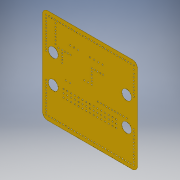
# Autodesk Inventor part: BaseBandAmp_Top_Bottom
Saved by Autodesk Inventor 2018 (Build 220112000, 112)
## iProperties
Created: 2018-03-27
Part Number: BaseBandAmp_Top_Bottom
Material: Generic
Document SubType Name: Modeling
Designer: Eric Weeks
Density: 1 g/cm^3
Appearance: Gold
Author: Eric Weeks
Autodesk Inventor part; units mm, degrees
ref_plane "YZ Plane" through (0, 0, 0) normal (1, 0, 0) x (0, 1, 0)
ref_plane "XZ Plane" through (0, 0, 0) normal (0, 1, 0) x (-1, 0, 0)
ref_plane "XY Plane" through (0, 0, 0) normal (0, 0, 1) x (1, 0, 0)
sketch "Sketch1" plane through (0, 0, 0) normal (0, 0, 1) x (1, 0, 0)
  circle A0 centre (3751.6054, -2038.7056) radius 4.8387 projected
  circle A1 centre (3732.2506, -2038.7056) radius 4.8387 projected
  circle A2 centre (3732.2506, -2038.7056) radius 4.8387 projected
  circle A3 centre (3712.8958, -2038.7056) radius 4.8387 projected
  circle A4 centre (3712.8958, -2038.7056) radius 4.8387 projected
  circle A5 centre (3693.541, -2038.7056) radius 4.8387 projected
  circle A6 centre (3693.541, -2038.7056) radius 4.8387 projected
  circle A7 centre (3674.1862, -2038.7056) radius 4.8387 projected
  circle A8 centre (3674.1862, -2038.7056) radius 4.8387 projected
  circle A9 centre (3751.6054, -2038.7056) radius 4.8387 projected
  line L0 (3839.1338, -1416.8501) -> (3850.1828, -1418.7957) projected
  line L1 (3850.1828, -1418.7957) -> (3850.9956, -1419.098) projected
  line L2 (3850.9956, -1419.098) -> (3860.6984, -1424.6987) projected
  line L3 (3860.6984, -1424.6987) -> (3861.0032, -1424.9425) projected
  line L4 (3861.0032, -1424.9425) -> (3861.3842, -1425.2651) projected
  line L5 (3861.3842, -1425.2651) -> (3868.5724, -1433.8478) projected
  line L6 (3868.5724, -1433.8478) -> (3869.0296, -1434.6123) projected
  line L7 (3869.0296, -1434.6123) -> (3872.865, -1445.1406) projected
  line L8 (3872.865, -1445.1406) -> (3872.9158, -1445.4657) projected
  line L9 (3872.9158, -1445.4657) -> (3872.992, -1445.7883) projected
  line L10 (3872.992, -1445.7883) -> (3873.5, -1451.389) projected
  line L11 (3873.5, -1451.389) -> (3873.4746, -1451.4627) projected
  line L12 (3873.4746, -1451.4627) -> (3873.5, -1451.5541) projected
  line L13 (3873.5, -1451.5541) -> (3873.5, -2032.3099) projected
  line L14 (3873.5, -2032.3099) -> (3873.4492, -2032.5283) projected
  line L15 (3873.4492, -2032.5283) -> (3873.4492, -2032.696) projected
  line L16 (3873.4492, -2032.696) -> (3871.5188, -2043.7272) projected
  line L17 (3871.5188, -2043.7272) -> (3871.214, -2044.5578) projected
  line L18 (3871.214, -2044.5578) -> (3865.6006, -2054.258) projected
  line L19 (3865.6006, -2054.258) -> (3865.0418, -2054.9337) projected
  line L20 (3865.0418, -2054.9337) -> (3856.4566, -2062.1371) projected
  line L21 (3856.4566, -2062.1371) -> (3855.6946, -2062.5765) projected
  line L22 (3855.6946, -2062.5765) -> (3845.179, -2066.4094) projected
  line L23 (3845.179, -2066.4094) -> (3844.8488, -2066.4653) projected
  line L24 (3844.8488, -2066.4653) -> (3844.5186, -2066.5516) projected
  line L25 (3844.5186, -2066.5516) -> (3838.9306, -2067.0418) projected
  line L26 (3838.9306, -2067.0418) -> (3838.8544, -2067.0368) projected
  line L27 (3838.8544, -2067.0368) -> (3838.7528, -2067.052) projected
  line L28 (3838.7528, -2067.052) -> (3258.0072, -2067.052) projected
  line L29 (3258.0072, -2067.052) -> (3257.7786, -2067.0139) projected
  line L30 (3257.7786, -2067.0139) -> (3257.6262, -2067.0139) projected
  line L31 (3257.6262, -2067.0139) -> (3246.5772, -2065.0683) projected
  line L32 (3246.5772, -2065.0683) -> (3245.7644, -2064.766) projected
  line L33 (3245.7644, -2064.766) -> (3236.0616, -2059.1653) projected
  line L34 (3236.0616, -2059.1653) -> (3235.7568, -2058.9215) projected
  line L35 (3235.7568, -2058.9215) -> (3235.3758, -2058.5989) projected
  line L36 (3235.3758, -2058.5989) -> (3228.1876, -2050.0162) projected
  line L37 (3228.1876, -2050.0162) -> (3227.7304, -2049.2517) projected
  line L38 (3227.7304, -2049.2517) -> (3223.895, -2038.7234) projected
  line L39 (3223.895, -2038.7234) -> (3223.8442, -2038.3983) projected
  line L40 (3223.8442, -2038.3983) -> (3223.768, -2038.0757) projected
  line L41 (3223.768, -2038.0757) -> (3223.26, -2032.475) projected
  line L42 (3223.26, -2032.475) -> (3223.2854, -2032.4013) projected
  line L43 (3223.2854, -2032.4013) -> (3223.26, -2032.3099) projected
  line L44 (3223.26, -2032.3099) -> (3223.26, -1451.5541) projected
  line L45 (3223.26, -1451.5541) -> (3223.3108, -1451.3357) projected
  line L46 (3223.3108, -1451.3357) -> (3223.3108, -1451.168) projected
  line L47 (3223.3108, -1451.168) -> (3225.2412, -1440.1368) projected
  line L48 (3225.2412, -1440.1368) -> (3225.546, -1439.3062) projected
  line L49 (3225.546, -1439.3062) -> (3231.1594, -1429.606) projected
  line L50 (3231.1594, -1429.606) -> (3231.4388, -1429.2682) projected
  line L51 (3231.4388, -1429.2682) -> (3231.7182, -1428.9303) projected
  line L52 (3231.7182, -1428.9303) -> (3240.3034, -1421.7269) projected
  line L53 (3240.3034, -1421.7269) -> (3241.0654, -1421.2875) projected
  line L54 (3241.0654, -1421.2875) -> (3251.581, -1417.4546) projected
  line L55 (3251.581, -1417.4546) -> (3251.9112, -1417.3987) projected
  line L56 (3251.9112, -1417.3987) -> (3252.2414, -1417.3124) projected
  line L57 (3252.2414, -1417.3124) -> (3257.8294, -1416.8222) projected
  line L58 (3257.8294, -1416.8222) -> (3257.9056, -1416.8272) projected
  line L59 (3257.9056, -1416.8272) -> (3258.0072, -1416.812) projected
  line L60 (3258.0072, -1416.812) -> (3838.7528, -1416.812) projected
  line L61 (3838.7528, -1416.812) -> (3838.9814, -1416.8501) projected
  line L62 (3838.9814, -1416.8501) -> (3839.1338, -1416.8501) projected
  circle A10 centre (3848.3794, -1470.9648) radius 4.8387 projected
  circle A11 centre (3848.3794, -1470.9648) radius 4.8387 projected
  circle A12 centre (3770.9602, -1445.1584) radius 4.8387 projected
  circle A13 centre (3770.9602, -1445.1584) radius 4.8387 projected
  circle A14 centre (3790.315, -1445.1584) radius 4.8387 projected
  circle A15 centre (3790.315, -1445.1584) radius 4.8387 projected
  circle A16 centre (3809.6698, -1445.1584) radius 4.8387 projected
  circle A17 centre (3809.6698, -1445.1584) radius 4.8387 projected
  circle A18 centre (3848.3794, -1445.1584) radius 4.8387 projected
  circle A19 centre (3848.3794, -1445.1584) radius 4.8387 projected
  circle A20 centre (3829.0246, -1445.1584) radius 4.8387 projected
  circle A21 centre (3829.0246, -1445.1584) radius 4.8387 projected
  circle A22 centre (3848.3794, -1593.5452) radius 4.8387 projected
  circle A23 centre (3848.3794, -1593.5452) radius 4.8387 projected
  circle A24 centre (3848.3794, -1612.9) radius 4.8387 projected
  circle A25 centre (3848.3794, -1612.9) radius 4.8387 projected
  circle A26 centre (3848.3794, -1632.2548) radius 4.8387 projected
  circle A27 centre (3848.3794, -1632.2548) radius 4.8387 projected
  circle A28 centre (3799.9924, -1645.158) radius 33.8709 projected
  circle A29 centre (3777.4118, -1783.8674) radius 4.8387 projected
  circle A30 centre (3799.9924, -1645.158) radius 33.8709 projected
  circle A31 centre (3848.3794, -1574.1904) radius 4.8387 projected
  circle A32 centre (3561.2832, -1606.4484) radius 4.8387 projected
  circle A33 centre (3580.638, -1606.4484) radius 4.8387 projected
  circle A34 centre (3599.9928, -1606.4484) radius 4.8387 projected
  circle A35 centre (3619.3476, -1606.4484) radius 4.8387 projected
  circle A36 centre (3638.7024, -1606.4484) radius 4.8387 projected
  circle A37 centre (3480.6382, -1445.1584) radius 4.8387 projected
  circle A38 centre (3499.993, -1445.1584) radius 4.8387 projected
  circle A39 centre (3635.4766, -1445.1584) radius 4.8387 projected
  circle A40 centre (3635.4766, -1445.1584) radius 4.8387 projected
  circle A41 centre (3616.1218, -1445.1584) radius 4.8387 projected
  circle A42 centre (3616.1218, -1445.1584) radius 4.8387 projected
  circle A43 centre (3638.7024, -1606.4484) radius 4.8387 projected
  circle A44 centre (3635.4766, -1548.384) radius 4.8387 projected
  circle A45 centre (3596.767, -1445.1584) radius 4.8387 projected
  circle A46 centre (3577.4122, -1445.1584) radius 4.8387 projected
  circle A47 centre (3577.4122, -1445.1584) radius 4.8387 projected
  circle A48 centre (3606.4444, -1548.384) radius 4.8387 projected
  circle A49 centre (3558.0574, -1445.1584) radius 4.8387 projected
  circle A50 centre (3558.0574, -1445.1584) radius 4.8387 projected
  circle A51 centre (3577.4122, -1548.384) radius 4.8387 projected
  circle A52 centre (3548.38, -1548.384) radius 4.8387 projected
  circle A53 centre (3538.7026, -1445.1584) radius 4.8387 projected
  circle A54 centre (3538.7026, -1445.1584) radius 4.8387 projected
  circle A55 centre (3519.3478, -1445.1584) radius 4.8387 projected
  circle A56 centre (3519.3478, -1445.1584) radius 4.8387 projected
  circle A57 centre (3499.993, -1445.1584) radius 4.8387 projected
  circle A58 centre (3480.6382, -1445.1584) radius 4.8387 projected
  circle A59 centre (3596.767, -1445.1584) radius 4.8387 projected
  circle A60 centre (3248.3806, -1464.5132) radius 4.8387 projected
  circle A61 centre (3248.3806, -1483.868) radius 4.8387 projected
  circle A62 centre (3248.3806, -1503.2228) radius 4.8387 projected
  circle A63 centre (3248.3806, -1522.5776) radius 4.8387 projected
  circle A64 centre (3312.8966, -1464.5132) radius 4.8387 projected
  circle A65 centre (3312.8966, -1464.5132) radius 4.8387 projected
  circle A66 centre (3248.3806, -1483.868) radius 4.8387 projected
  circle A67 centre (3248.3806, -1464.5132) radius 4.8387 projected
  circle A68 centre (3248.3806, -1503.2228) radius 4.8387 projected
  circle A69 centre (3248.3806, -1522.5776) radius 4.8387 projected
  circle A70 centre (3248.3806, -1580.642) radius 4.8387 projected
  circle A71 centre (3248.3806, -1580.642) radius 4.8387 projected
  circle A72 centre (3248.3806, -1561.2872) radius 4.8387 projected
  circle A73 centre (3248.3806, -1561.2872) radius 4.8387 projected
  circle A74 centre (3248.3806, -1541.9324) radius 4.8387 projected
  circle A75 centre (3248.3806, -1541.9324) radius 4.8387 projected
  circle A76 centre (3248.3806, -1832.2544) radius 4.8387 projected
  circle A77 centre (3248.3806, -1967.738) radius 4.8387 projected
  circle A78 centre (3248.3806, -1948.3832) radius 4.8387 projected
  circle A79 centre (3248.3806, -1948.3832) radius 4.8387 projected
  circle A80 centre (3248.3806, -1929.0284) radius 4.8387 projected
  circle A81 centre (3248.3806, -1929.0284) radius 4.8387 projected
  circle A82 centre (3248.3806, -1909.6736) radius 4.8387 projected
  circle A83 centre (3248.3806, -1909.6736) radius 4.8387 projected
  circle A84 centre (3248.3806, -1890.3188) radius 4.8387 projected
  circle A85 centre (3248.3806, -1890.3188) radius 4.8387 projected
  circle A86 centre (3248.3806, -1870.964) radius 4.8387 projected
  circle A87 centre (3248.3806, -1870.964) radius 4.8387 projected
  circle A88 centre (3248.3806, -1851.6092) radius 4.8387 projected
  circle A89 centre (3248.3806, -1851.6092) radius 4.8387 projected
  circle A90 centre (3248.3806, -1832.2544) radius 4.8387 projected
  circle A91 centre (3296.7676, -1838.706) radius 33.8709 projected
  circle A92 centre (3296.7676, -1838.706) radius 33.8709 projected
  circle A93 centre (3248.3806, -1967.738) radius 4.8387 projected
  circle A94 centre (3848.3794, -1961.2864) radius 4.8387 projected
  circle A95 centre (3848.3794, -1941.9316) radius 4.8387 projected
  circle A96 centre (3848.3794, -1922.5768) radius 4.8387 projected
  circle A97 centre (3848.3794, -1903.222) radius 4.8387 projected
  circle A98 centre (3848.3794, -1883.8672) radius 4.8387 projected
  circle A99 centre (3848.3794, -1864.5124) radius 4.8387 projected
  circle A100 centre (3848.3794, -1845.1576) radius 4.8387 projected
  circle A101 centre (3848.3794, -1825.8028) radius 4.8387 projected
  circle A102 centre (3651.6056, -1825.8028) radius 4.8387 projected
  circle A103 centre (3677.412, -1825.8028) radius 4.8387 projected
  circle A104 centre (3677.412, -1877.4156) radius 4.8387 projected
  circle A105 centre (3703.2184, -1877.4156) radius 4.8387 projected
  circle A106 centre (3729.0248, -1877.4156) radius 4.8387 projected
  circle A107 centre (3651.6056, -1877.4156) radius 4.8387 projected
  circle A108 centre (3651.6056, -1851.6092) radius 4.8387 projected
  circle A109 centre (3677.412, -1851.6092) radius 4.8387 projected
  circle A110 centre (3848.3794, -1941.9316) radius 4.8387 projected
  circle A111 centre (3848.3794, -1922.5768) radius 4.8387 projected
  circle A112 centre (3703.2184, -1851.6092) radius 4.8387 projected
  circle A113 centre (3729.0248, -1851.6092) radius 4.8387 projected
  circle A114 centre (3703.2184, -1825.8028) radius 4.8387 projected
  circle A115 centre (3729.0248, -1825.8028) radius 4.8387 projected
  circle A116 centre (3848.3794, -1903.222) radius 4.8387 projected
  circle A117 centre (3848.3794, -1883.8672) radius 4.8387 projected
  circle A118 centre (3848.3794, -1864.5124) radius 4.8387 projected
  circle A119 centre (3799.9924, -1838.706) radius 33.8709 projected
  circle A120 centre (3799.9924, -1838.706) radius 33.8709 projected
  circle A121 centre (3848.3794, -1845.1576) radius 4.8387 projected
  circle A122 centre (3848.3794, -1825.8028) radius 4.8387 projected
  circle A123 centre (3848.3794, -1961.2864) radius 4.8387 projected
  circle A124 centre (3770.9602, -2038.7056) radius 4.8387 projected
  circle A125 centre (3790.315, -2038.7056) radius 4.8387 projected
  circle A126 centre (3790.315, -2038.7056) radius 4.8387 projected
  circle A127 centre (3809.6698, -2038.7056) radius 4.8387 projected
  circle A128 centre (3809.6698, -2038.7056) radius 4.8387 projected
  circle A129 centre (3829.0246, -2038.7056) radius 4.8387 projected
  circle A130 centre (3829.0246, -2038.7056) radius 4.8387 projected
  circle A131 centre (3848.3794, -1980.6412) radius 4.8387 projected
  circle A132 centre (3848.3794, -1980.6412) radius 4.8387 projected
  circle A133 centre (3848.3794, -1999.996) radius 4.8387 projected
  circle A134 centre (3848.3794, -1999.996) radius 4.8387 projected
  circle A135 centre (3848.3794, -2019.3508) radius 4.8387 projected
  circle A136 centre (3848.3794, -2019.3508) radius 4.8387 projected
  circle A137 centre (3848.3794, -2038.7056) radius 4.8387 projected
  circle A138 centre (3848.3794, -2038.7056) radius 4.8387 projected
  circle A139 centre (3770.9602, -2038.7056) radius 4.8387 projected
  circle A140 centre (3383.8642, -1767.7384) radius 4.8387 projected
  circle A141 centre (3412.8964, -1767.7384) radius 4.8387 projected
  circle A142 centre (3367.7352, -1825.8028) radius 4.8387 projected
  circle A143 centre (3393.5416, -1825.8028) radius 4.8387 projected
  circle A144 centre (3419.348, -1825.8028) radius 4.8387 projected
  circle A145 centre (3367.7352, -1851.6092) radius 4.8387 projected
  circle A146 centre (3393.5416, -1851.6092) radius 4.8387 projected
  circle A147 centre (3419.348, -1851.6092) radius 4.8387 projected
  circle A148 centre (3419.348, -1877.4156) radius 4.8387 projected
  circle A149 centre (3419.348, -1877.4156) radius 4.8387 projected
  circle A150 centre (3419.348, -1825.8028) radius 4.8387 projected
  circle A151 centre (3393.5416, -1877.4156) radius 4.8387 projected
  circle A152 centre (3393.5416, -1877.4156) radius 4.8387 projected
  circle A153 centre (3393.5416, -1851.6092) radius 4.8387 projected
  circle A154 centre (3393.5416, -1825.8028) radius 4.8387 projected
  circle A155 centre (3367.7352, -1877.4156) radius 4.8387 projected
  circle A156 centre (3367.7352, -1877.4156) radius 4.8387 projected
  circle A157 centre (3412.8964, -1767.7384) radius 4.8387 projected
  circle A158 centre (3367.7352, -1851.6092) radius 4.8387 projected
  circle A159 centre (3367.7352, -1825.8028) radius 4.8387 projected
  circle A160 centre (3383.8642, -1767.7384) radius 4.8387 projected
  circle A161 centre (3419.348, -1851.6092) radius 4.8387 projected
  circle A162 centre (3558.0574, -2038.7056) radius 4.8387 projected
  circle A163 centre (3577.4122, -2038.7056) radius 4.8387 projected
  circle A164 centre (3596.767, -2038.7056) radius 4.8387 projected
  circle A165 centre (3616.1218, -2038.7056) radius 4.8387 projected
  circle A166 centre (3635.4766, -2038.7056) radius 4.8387 projected
  circle A167 centre (3635.4766, -2038.7056) radius 4.8387 projected
  circle A168 centre (3596.767, -2038.7056) radius 4.8387 projected
  circle A169 centre (3577.4122, -2038.7056) radius 4.8387 projected
  circle A170 centre (3558.0574, -2038.7056) radius 4.8387 projected
  circle A171 centre (3616.1218, -2038.7056) radius 4.8387 projected
  circle A172 centre (3758.057, -1783.8674) radius 4.8387 projected
  circle A173 centre (3777.4118, -1783.8674) radius 4.8387 projected
  circle A174 centre (3799.9924, -1783.8674) radius 4.8387 projected
  circle A175 centre (3758.057, -1783.8674) radius 4.8387 projected
  circle A176 centre (3799.9924, -1783.8674) radius 4.8387 projected
  circle A177 centre (3248.3806, -1599.9968) radius 4.8387 projected
  circle A178 centre (3248.3806, -1619.3516) radius 4.8387 projected
  circle A179 centre (3248.3806, -1638.7064) radius 4.8387 projected
  circle A180 centre (3248.3806, -1658.0612) radius 4.8387 projected
  circle A181 centre (3358.0578, -1677.416) radius 4.8387 projected
  circle A182 centre (3358.0578, -1658.0612) radius 4.8387 projected
  circle A183 centre (3358.0578, -1638.7064) radius 4.8387 projected
  circle A184 centre (3358.0578, -1619.3516) radius 4.8387 projected
  circle A185 centre (3358.0578, -1599.9968) radius 4.8387 projected
  circle A186 centre (3358.0578, -1599.9968) radius 4.8387 projected
  circle A187 centre (3248.3806, -1599.9968) radius 4.8387 projected
  circle A188 centre (3248.3806, -1619.3516) radius 4.8387 projected
  circle A189 centre (3358.0578, -1619.3516) radius 4.8387 projected
  circle A190 centre (3248.3806, -1638.7064) radius 4.8387 projected
  circle A191 centre (3248.3806, -1658.0612) radius 4.8387 projected
  circle A192 centre (3296.7676, -1645.158) radius 33.8709 projected
  circle A193 centre (3296.7676, -1645.158) radius 33.8709 projected
  circle A194 centre (3358.0578, -1658.0612) radius 4.8387 projected
  circle A195 centre (3358.0578, -1677.416) radius 4.8387 projected
  circle A196 centre (3358.0578, -1638.7064) radius 4.8387 projected
  circle A197 centre (3332.2514, -1599.9968) radius 4.8387 projected
  circle A198 centre (3654.8314, -1445.1584) radius 4.8387 projected
  circle A199 centre (3654.8314, -1445.1584) radius 4.8387 projected
  circle A200 centre (3674.1862, -1445.1584) radius 4.8387 projected
  circle A201 centre (3674.1862, -1445.1584) radius 4.8387 projected
  circle A202 centre (3693.541, -1445.1584) radius 4.8387 projected
  circle A203 centre (3712.8958, -1445.1584) radius 4.8387 projected
  circle A204 centre (3712.8958, -1445.1584) radius 4.8387 projected
  circle A205 centre (3732.2506, -1445.1584) radius 4.8387 projected
  circle A206 centre (3732.2506, -1445.1584) radius 4.8387 projected
  circle A207 centre (3751.6054, -1445.1584) radius 4.8387 projected
  circle A208 centre (3751.6054, -1445.1584) radius 4.8387 projected
  circle A209 centre (3693.541, -1445.1584) radius 4.8387 projected
  circle A210 centre (3312.8966, -1564.513) radius 4.8387 projected
  circle A211 centre (3312.8966, -1545.1582) radius 4.8387 projected
  circle A212 centre (3312.8966, -1525.8034) radius 4.8387 projected
  circle A213 centre (3312.8966, -1506.4486) radius 4.8387 projected
  circle A214 centre (3312.8966, -1564.513) radius 4.8387 projected
  circle A215 centre (3312.8966, -1545.1582) radius 4.8387 projected
  circle A216 centre (3312.8966, -1525.8034) radius 4.8387 projected
  circle A217 centre (3312.8966, -1506.4486) radius 4.8387 projected
  circle A218 centre (3312.8966, -1487.0938) radius 4.8387 projected
  circle A219 centre (3312.8966, -1587.0936) radius 4.8387 projected
  circle A220 centre (3312.8966, -1587.0936) radius 4.8387 projected
  circle A221 centre (3332.2514, -1599.9968) radius 4.8387 projected
  circle A222 centre (3377.4126, -1599.9968) radius 4.8387 projected
  circle A223 centre (3377.4126, -1599.9968) radius 4.8387 projected
  circle A224 centre (3396.7674, -1599.9968) radius 4.8387 projected
  circle A225 centre (3396.7674, -1599.9968) radius 4.8387 projected
  circle A226 centre (3416.1222, -1599.9968) radius 4.8387 projected
  circle A227 centre (3416.1222, -1599.9968) radius 4.8387 projected
  circle A228 centre (3412.8964, -1545.1582) radius 4.8387 projected
  circle A229 centre (3412.8964, -1545.1582) radius 4.8387 projected
  circle A230 centre (3312.8966, -1487.0938) radius 4.8387 projected
  circle A231 centre (3445.1544, -1825.8028) radius 4.8387 projected
  circle A232 centre (3470.9608, -1825.8028) radius 4.8387 projected
  circle A233 centre (3496.7672, -1825.8028) radius 4.8387 projected
  circle A234 centre (3522.5736, -1825.8028) radius 4.8387 projected
  circle A235 centre (3548.38, -1825.8028) radius 4.8387 projected
  circle A236 centre (3445.1544, -1851.6092) radius 4.8387 projected
  circle A237 centre (3470.9608, -1851.6092) radius 4.8387 projected
  circle A238 centre (3496.7672, -1851.6092) radius 4.8387 projected
  circle A239 centre (3522.5736, -1851.6092) radius 4.8387 projected
  circle A240 centre (3445.1544, -1877.4156) radius 4.8387 projected
  circle A241 centre (3445.1544, -1825.8028) radius 4.8387 projected
  circle A242 centre (3445.1544, -1851.6092) radius 4.8387 projected
  circle A243 centre (3470.9608, -1877.4156) radius 4.8387 projected
  circle A244 centre (3470.9608, -1877.4156) radius 4.8387 projected
  circle A245 centre (3470.9608, -1851.6092) radius 4.8387 projected
  circle A246 centre (3470.9608, -1825.8028) radius 4.8387 projected
  circle A247 centre (3496.7672, -1825.8028) radius 4.8387 projected
  circle A248 centre (3496.7672, -1851.6092) radius 4.8387 projected
  circle A249 centre (3496.7672, -1877.4156) radius 4.8387 projected
  circle A250 centre (3496.7672, -1877.4156) radius 4.8387 projected
  circle A251 centre (3522.5736, -1851.6092) radius 4.8387 projected
  circle A252 centre (3522.5736, -1877.4156) radius 4.8387 projected
  circle A253 centre (3522.5736, -1877.4156) radius 4.8387 projected
  circle A254 centre (3548.38, -1851.6092) radius 4.8387 projected
  circle A255 centre (3548.38, -1851.6092) radius 4.8387 projected
  circle A256 centre (3548.38, -1877.4156) radius 4.8387 projected
  circle A257 centre (3548.38, -1877.4156) radius 4.8387 projected
  circle A258 centre (3445.1544, -1877.4156) radius 4.8387 projected
  circle A259 centre (3345.1546, -2038.7056) radius 4.8387 projected
  circle A260 centre (3364.5094, -2038.7056) radius 4.8387 projected
  circle A261 centre (3383.8642, -2038.7056) radius 4.8387 projected
  circle A262 centre (3403.219, -2038.7056) radius 4.8387 projected
  circle A263 centre (3422.5738, -2038.7056) radius 4.8387 projected
  circle A264 centre (3441.9286, -2038.7056) radius 4.8387 projected
  circle A265 centre (3461.2834, -2038.7056) radius 4.8387 projected
  circle A266 centre (3480.6382, -2038.7056) radius 4.8387 projected
  circle A267 centre (3499.993, -2038.7056) radius 4.8387 projected
  circle A268 centre (3519.3478, -2038.7056) radius 4.8387 projected
  circle A269 centre (3538.7026, -2038.7056) radius 4.8387 projected
  circle A270 centre (3345.1546, -2038.7056) radius 4.8387 projected
  circle A271 centre (3364.5094, -2038.7056) radius 4.8387 projected
  circle A272 centre (3383.8642, -2038.7056) radius 4.8387 projected
  circle A273 centre (3403.219, -2038.7056) radius 4.8387 projected
  circle A274 centre (3422.5738, -2038.7056) radius 4.8387 projected
  circle A275 centre (3441.9286, -2038.7056) radius 4.8387 projected
  circle A276 centre (3461.2834, -2038.7056) radius 4.8387 projected
  circle A277 centre (3480.6382, -2038.7056) radius 4.8387 projected
  circle A278 centre (3499.993, -2038.7056) radius 4.8387 projected
  circle A279 centre (3519.3478, -2038.7056) radius 4.8387 projected
  circle A280 centre (3538.7026, -2038.7056) radius 4.8387 projected
  circle A281 centre (3654.8314, -2038.7056) radius 4.8387 projected
  circle A282 centre (3654.8314, -2038.7056) radius 4.8387 projected
  circle A283 centre (3641.9282, -1783.8674) radius 4.8387 projected
  circle A284 centre (3661.283, -1783.8674) radius 4.8387 projected
  circle A285 centre (3680.6378, -1783.8674) radius 4.8387 projected
  circle A286 centre (3699.9926, -1783.8674) radius 4.8387 projected
  circle A287 centre (3719.3474, -1783.8674) radius 4.8387 projected
  circle A288 centre (3738.7022, -1783.8674) radius 4.8387 projected
  circle A289 centre (3738.7022, -1783.8674) radius 4.8387 projected
  circle A290 centre (3729.0248, -1825.8028) radius 4.8387 projected
  circle A291 centre (3729.0248, -1851.6092) radius 4.8387 projected
  circle A292 centre (3729.0248, -1877.4156) radius 4.8387 projected
  circle A293 centre (3719.3474, -1783.8674) radius 4.8387 projected
  circle A294 centre (3703.2184, -1825.8028) radius 4.8387 projected
  circle A295 centre (3703.2184, -1851.6092) radius 4.8387 projected
  circle A296 centre (3703.2184, -1877.4156) radius 4.8387 projected
  circle A297 centre (3699.9926, -1783.8674) radius 4.8387 projected
  circle A298 centre (3680.6378, -1783.8674) radius 4.8387 projected
  circle A299 centre (3677.412, -1825.8028) radius 4.8387 projected
  circle A300 centre (3677.412, -1851.6092) radius 4.8387 projected
  circle A301 centre (3677.412, -1877.4156) radius 4.8387 projected
  circle A302 centre (3651.6056, -1877.4156) radius 4.8387 projected
  circle A303 centre (3661.283, -1783.8674) radius 4.8387 projected
  circle A304 centre (3641.9282, -1783.8674) radius 4.8387 projected
  circle A305 centre (3651.6056, -1825.8028) radius 4.8387 projected
  circle A306 centre (3651.6056, -1851.6092) radius 4.8387 projected
  circle A307 centre (3603.2186, -1783.8674) radius 4.8387 projected
  circle A308 centre (3622.5734, -1783.8674) radius 4.8387 projected
  circle A309 centre (3574.1864, -1825.8028) radius 4.8387 projected
  circle A310 centre (3599.9928, -1825.8028) radius 4.8387 projected
  circle A311 centre (3625.7992, -1825.8028) radius 4.8387 projected
  circle A312 centre (3574.1864, -1851.6092) radius 4.8387 projected
  circle A313 centre (3599.9928, -1851.6092) radius 4.8387 projected
  circle A314 centre (3625.7992, -1851.6092) radius 4.8387 projected
  circle A315 centre (3574.1864, -1877.4156) radius 4.8387 projected
  circle A316 centre (3599.9928, -1877.4156) radius 4.8387 projected
  circle A317 centre (3625.7992, -1877.4156) radius 4.8387 projected
  circle A318 centre (3603.2186, -1783.8674) radius 4.8387 projected
  circle A319 centre (3622.5734, -1783.8674) radius 4.8387 projected
  circle A320 centre (3625.7992, -1825.8028) radius 4.8387 projected
  circle A321 centre (3625.7992, -1851.6092) radius 4.8387 projected
  circle A322 centre (3625.7992, -1877.4156) radius 4.8387 projected
  circle A323 centre (3599.9928, -1825.8028) radius 4.8387 projected
  circle A324 centre (3599.9928, -1851.6092) radius 4.8387 projected
  circle A325 centre (3599.9928, -1877.4156) radius 4.8387 projected
  circle A326 centre (3574.1864, -1825.8028) radius 4.8387 projected
  circle A327 centre (3574.1864, -1851.6092) radius 4.8387 projected
  circle A328 centre (3574.1864, -1877.4156) radius 4.8387 projected
  circle A329 centre (3522.5736, -1825.8028) radius 4.8387 projected
  circle A330 centre (3548.38, -1825.8028) radius 4.8387 projected
  circle A331 centre (3561.2832, -1625.8032) radius 4.8387 projected
  circle A332 centre (3561.2832, -1645.158) radius 4.8387 projected
  circle A333 centre (3561.2832, -1664.5128) radius 4.8387 projected
  circle A334 centre (3561.2832, -1683.8676) radius 4.8387 projected
  circle A335 centre (3561.2832, -1703.2224) radius 4.8387 projected
  circle A336 centre (3535.4768, -1703.2224) radius 4.8387 projected
  circle A337 centre (3509.6704, -1703.2224) radius 4.8387 projected
  circle A338 centre (3561.2832, -1606.4484) radius 4.8387 projected
  circle A339 centre (3580.638, -1606.4484) radius 4.8387 projected
  circle A340 centre (3599.9928, -1606.4484) radius 4.8387 projected
  circle A341 centre (3619.3476, -1606.4484) radius 4.8387 projected
  circle A342 centre (3561.2832, -1625.8032) radius 4.8387 projected
  circle A343 centre (3561.2832, -1645.158) radius 4.8387 projected
  circle A344 centre (3561.2832, -1664.5128) radius 4.8387 projected
  circle A345 centre (3561.2832, -1703.2224) radius 4.8387 projected
  circle A346 centre (3561.2832, -1683.8676) radius 4.8387 projected
  circle A347 centre (3509.6704, -1703.2224) radius 4.8387 projected
  circle A348 centre (3635.4766, -1548.384) radius 4.8387 projected
  circle A349 centre (3606.4444, -1548.384) radius 4.8387 projected
  circle A350 centre (3577.4122, -1548.384) radius 4.8387 projected
  circle A351 centre (3548.38, -1548.384) radius 4.8387 projected
  circle A352 centre (3535.4768, -1703.2224) radius 4.8387 projected
  circle A353 centre (3848.3794, -1496.7712) radius 4.8387 projected
  circle A354 centre (3848.3794, -1496.7712) radius 4.8387 projected
  circle A355 centre (3848.3794, -1516.126) radius 4.8387 projected
  circle A356 centre (3848.3794, -1516.126) radius 4.8387 projected
  circle A357 centre (3848.3794, -1535.4808) radius 4.8387 projected
  circle A358 centre (3848.3794, -1535.4808) radius 4.8387 projected
  circle A359 centre (3848.3794, -1554.8356) radius 4.8387 projected
  circle A360 centre (3848.3794, -1574.1904) radius 4.8387 projected
  circle A361 centre (3848.3794, -1554.8356) radius 4.8387 projected
  circle A362 centre (3248.3806, -1987.0928) radius 4.8387 projected
  circle A363 centre (3248.3806, -2006.4476) radius 4.8387 projected
  circle A364 centre (3248.3806, -2006.4476) radius 4.8387 projected
  circle A365 centre (3248.3806, -2022.5766) radius 4.8387 projected
  circle A366 centre (3248.3806, -2022.5766) radius 4.8387 projected
  circle A367 centre (3325.7998, -2038.7056) radius 4.8387 projected
  circle A368 centre (3325.7998, -2038.7056) radius 4.8387 projected
  circle A369 centre (3306.445, -2038.7056) radius 4.8387 projected
  circle A370 centre (3306.445, -2038.7056) radius 4.8387 projected
  circle A371 centre (3287.0902, -2038.7056) radius 4.8387 projected
  circle A372 centre (3287.0902, -2038.7056) radius 4.8387 projected
  circle A373 centre (3267.7354, -2038.7056) radius 4.8387 projected
  circle A374 centre (3267.7354, -2038.7056) radius 4.8387 projected
  circle A375 centre (3248.3806, -2038.7056) radius 4.8387 projected
  circle A376 centre (3248.3806, -2038.7056) radius 4.8387 projected
  circle A377 centre (3248.3806, -1987.0928) radius 4.8387 projected
  circle A378 centre (3248.3806, -1445.1584) radius 4.8387 projected
  circle A379 centre (3267.7354, -1445.1584) radius 4.8387 projected
  circle A380 centre (3287.0902, -1445.1584) radius 4.8387 projected
  circle A381 centre (3306.445, -1445.1584) radius 4.8387 projected
  circle A382 centre (3325.7998, -1445.1584) radius 4.8387 projected
  circle A383 centre (3345.1546, -1445.1584) radius 4.8387 projected
  circle A384 centre (3364.5094, -1445.1584) radius 4.8387 projected
  circle A385 centre (3383.8642, -1445.1584) radius 4.8387 projected
  circle A386 centre (3403.219, -1445.1584) radius 4.8387 projected
  circle A387 centre (3422.5738, -1445.1584) radius 4.8387 projected
  circle A388 centre (3441.9286, -1445.1584) radius 4.8387 projected
  circle A389 centre (3461.2834, -1445.1584) radius 4.8387 projected
  circle A390 centre (3438.7028, -1545.1582) radius 4.8387 projected
  circle A391 centre (3467.735, -1545.1582) radius 4.8387 projected
  circle A392 centre (3248.3806, -1445.1584) radius 4.8387 projected
  circle A393 centre (3267.7354, -1445.1584) radius 4.8387 projected
  circle A394 centre (3287.0902, -1445.1584) radius 4.8387 projected
  circle A395 centre (3306.445, -1445.1584) radius 4.8387 projected
  circle A396 centre (3325.7998, -1445.1584) radius 4.8387 projected
  circle A397 centre (3345.1546, -1445.1584) radius 4.8387 projected
  circle A398 centre (3364.5094, -1445.1584) radius 4.8387 projected
  circle A399 centre (3383.8642, -1445.1584) radius 4.8387 projected
  circle A400 centre (3403.219, -1445.1584) radius 4.8387 projected
  circle A401 centre (3422.5738, -1445.1584) radius 4.8387 projected
  circle A402 centre (3438.7028, -1545.1582) radius 4.8387 projected
  circle A403 centre (3467.735, -1545.1582) radius 4.8387 projected
  circle A404 centre (3461.2834, -1445.1584) radius 4.8387 projected
  circle A405 centre (3441.9286, -1445.1584) radius 4.8387 projected
  point P0 (0, 0)
extrude "Extrusion1" add sketch "Sketch1" along normal blind 0.9032
body "Solid1"
